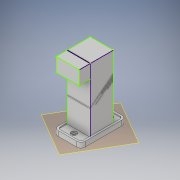
# Autodesk Inventor part: detector curvament fil
Saved by Autodesk Inventor 2019 (Build 230136000, 136)
## iProperties
Created: 2018-08-06
Part Number: detector curvament fil
Material: Genérico
Document SubType Name: Modeling
Designer: Albert Garangou Culebras
Density: 1 g/cm^3
Appearance: Valor por defecto
Mass: 54.1896 g
Surface Area: 120.446 cm^2
Volume: 54.1896 cm^3
Author: Albert Garangou Culebras
Title: suport detector curvament fil
Comments: Falta fer una possible guia per amagar el cable (dins la paret o a fora).
Autodesk Inventor part; units mm, degrees
ref_plane "YZ Plane" through (0, 0, 0) normal (1, 0, 0) x (0, 1, 0)
ref_plane "XZ Plane" through (0, 0, 0) normal (0, 1, 0) x (-1, 0, 0)
ref_plane "XY Plane" through (0, 0, 0) normal (0, 0, 1) x (1, 0, 0)
sketch3d "estructura"
sketch "base" plane through (0, 0, 0) normal (0, 1, 0) x (-1, 0, 0)
  line L0 (25, 0) -> (25, -25)
  line L1 (25, -25) -> (0, -25)
  line L2 (0, -25) -> (0, 0)
  line L3 (0, 0) -> (25, 0)
  line L4 (25, 0) -> (0, 0)
  line L5 (0, 0) -> (0, -25)
  line L6 (0, -25) -> (25, -25)
  line L7 (25, -25) -> (25, 0)
  constraints: 16 end point, 3 parallel, 1 horizontal, 1 perpendicular
sketch "Boceto4" plane through (0, 0, 0) normal (0, 0, 1) x (1, 0, 0)
  line L0 (-25, 75) -> (0, 75)
  line L1 (0, 75) -> (0, 60)
  line L2 (0, 60) -> (-25, 60)
  line L3 (-25, 60) -> (-25, 75)
  line L4 (-25, 75) -> (0, 75)
  point P0 (0, 0)
  constraints: 10 end point, 3 equal length, 1 horizontal, 1 perpendicular
extrude "suport" add sketch "Boceto4" along normal blind 12
extrude "cos" add sketch "base" along normal blind 75
sketch "borera" plane through (0, 0, 0) normal (0, -1, 0) x (1, 0, 0)
  line L0 (-25, -37) -> (0, -37)
  line L1 (-25, -25) -> (-25, 0) projected
  line L2 (0, 12) -> (-25, 12)
  line L3 (3, -24) -> (3, -37)
  line L4 (3, -37) -> (0, -37)
  line L5 (0, 12) -> (3, 12)
  line L6 (3, 12) -> (3, -24)
  line L7 (-25, -37) -> (-28, -37)
  line L8 (-25, 12) -> (-28, 12)
  line L9 (-28, 12) -> (-28, -37)
  point P0 (0, 0)
  point P1 (-25, -24)
  constraints: 18 end point, 3 horizontal, 2 perpendicular
extrude "borera?" add sketch "borera" against normal blind 7.5
sketch "LLOSA" plane through (0, 7.5, 0) normal (0, 1, 0) x (1, 0, 0)
  line L0 (0, -10) -> (-25, -10)
  line L1 (0, 35) -> (-25, 35)
  line L2 (0, -10) -> (0, 35)
  line L3 (-25, -10) -> (-25, 35)
  point P0 (0, 0)
  constraints: 8 end point, 1 perpendicular
sketch "Boceto7" plane through (3, 0, 12) normal (1, 0, 0) x (0, 0, -1)
  line L0 (0, 7.5) -> (49, 7.5)
  line L1 (49, 7.5) -> (49, 0)
  line L2 (49, 0) -> (0, 0)
  line L3 (0, 0) -> (0, 7.5)
  point P0 (12, 0)
  constraints: 8 end point, 2 parallel, 1 horizontal, 1 perpendicular
extrude "redimensió costat 2" cut sketch "Boceto7" against normal blind 1
sketch "Boceto8" plane through (-28, 0, -37) normal (-1, 0, 0) x (0, 0, 1)
  line L0 (49, 0) -> (49, 7.5) projected
  line L1 (0, 0) -> (0, 7.5) projected
  line L2 (49, 7.5) -> (0, 7.5)
  line L3 (0, 7.5) -> (0, 0)
  line L4 (0, 0) -> (49, 0)
  line L5 (49, 0) -> (49, 7.5)
  point P0 (37, 0)
  constraints: 8 end point, 2 parallel, 1 horizontal, 1 perpendicular
extrude "redimensió costat" cut sketch "Boceto8" against normal blind 1
extrude "foradar interior borera" cut sketch "LLOSA" against normal blind 1
sketch "rodons interns" plane through (0, 7.5, 0) normal (0, 1, 0) x (1, 0, 0)
  line L0 (-25, 35) -> (0, 35) projected
  line L1 (2, 35) -> (-2.5, 35)
  line L2 (-25, 35) -> (0, 35) projected
  line L3 (2, 37) -> (2, 32.5)
  line L4 (2, -12) -> (2, 37) projected
  circle A0 centre (-2.5, 32.5) radius 2.5
  circle A1 centre (-22.5, 32.5) radius 2.5
  line L5 (2, -12) -> (-2.5, -12)
  line L6 (-2.5, -12) -> (-2.5, -7.5)
  line L7 (-2.5, -7.5) -> (2, -7.5)
  line L8 (2, -7.5) -> (2, -12)
  line L9 (-27, -12) -> (-22.5, -12)
  line L10 (-22.5, -12) -> (-22.5, -7.5)
  line L11 (-22.5, -7.5) -> (-27, -7.5)
  line L12 (-27, -7.5) -> (-27, -12)
  circle A2 centre (-22.5, -7.5) radius 2.5
  line L13 (0, -10) -> (-25, -10) projected
  line L14 (-22.5, -10) -> (-25, -10)
  line L15 (-25, -10) -> (-25, -7.5)
  line L16 (-25, -10) -> (-25, 0) projected
  arc A3 (-25, -7.5) -> (-22.5, -10) centre (-22.5, -7.5) ccw
  circle A4 centre (-2.5, -7.5) radius 2.5
  arc A5 (-2.5, -10) -> (0, -7.5) centre (-2.5, -7.5) ccw
  line L17 (0, 0) -> (0, -10) projected
  line L18 (0, -7.5) -> (0, -10)
  line L19 (0, -10) -> (-2.5, -10)
  line L20 (-2.5, 35) -> (0, 35)
  line L21 (0, 35) -> (0, 25) projected
  arc A6 (0, 32.5) -> (-2.5, 35) centre (-2.5, 32.5) ccw
  arc A7 (-22.5, 35) -> (-25, 32.5) centre (-22.5, 32.5) ccw
  line L22 (-22.5, 35) -> (-25, 35)
  arc A8 (-22.5, 35) -> (-25, 32.5) centre (-22.5, 32.5) ccw
  line L23 (-25, 35) -> (-25, 32.5)
  line L24 (-25, 25) -> (-25, 35) projected
  arc A9 (-22.5, 35) -> (-25, 32.5) centre (-22.5, 32.5) ccw
  line L25 (-25, 32.5) -> (-25, 35)
  point P0 (-27, 37)
  dimension "d73" = 4.5
  dimension "d74" = 4.5
  dimension "d77" = 4.5
  dimension "d78" = 4.5
  constraints: 36 end point, 20 point on circle, 10 centre point, 7 tangent, 6 point on line, 5 collinear, 5 concentric, 4 parallel, 3 horizontal, 2 coincident, 2 perpendicular, 1 vertical
  measures "d73" distance of L1.start L1.end
  measures "d74" distance of L3.start L3.end
  measures "d77" distance of L6.end L7.end
  measures "d78" distance of L5.end L6.end
fillet "arrodoniment costats ext" radius 4.5 4 edges at (2, 3.75, -37) (-27, 3.75, -37) (2, 3.75, 12) (-27, 3.75, 12)
extrude "costats" add sketch "rodons interns" against normal blind 1 contours L0 A1 L23 | L0 L21 A0 | L17 L13 A4 | L13 L15 A2
sketch "cargols" plane through (0, 6.5, 0) normal (0, 1, 0) x (1, 0, 0)
  line L0 (0, 32.5) -> (0, 25) projected
  line L1 (-25, 25) -> (-25, 0) projected
  line L2 (-25, 0) -> (-25, -10)
  line L3 (-2.5, -10) -> (-22.5, -10) projected
  line L4 (-2.5, -10) -> (-25, -10)
  line L5 (-25, -7.5) -> (-25, 32.5) projected
  line L6 (0, 32.5) -> (0, -7.5) projected
  line L7 (-25, 25) -> (-25, 35.3997)
  line L8 (-22.5, 35) -> (-25, 35)
  line L9 (-25, 35) -> (-25, 25)
  circle A0 centre (-16.67, 30) radius 3
  circle A1 centre (-8.34, 30) radius 3
  line L10 (-25, -10) -> (-25, 0)
  circle A2 centre (-12.5, -5) radius 3
  point P0 (0, 0)
  dimension "d118" = 6
  dimension "d119" = 6
  dimension "d121" = 6
  constraints: 12 end point, 3 centre point, 3 vertical, 2 perpendicular, 2 point on line, 1 collinear
  measures "d118" diameter of A0
  measures "d119" diameter of A1
  measures "d121" diameter of A2
sketch "Boceto11" plane through (-25, 75, 12) normal (0, 1, 0) x (1, 0, 0)
  line L0 (0, 12) -> (25, 12) projected
  line L1 (25, 44.5) -> (25, 37) projected
  line L2 (0, 12) -> (25, 12)
  line L3 (25, 12) -> (25, 37)
  line L4 (25, 37) -> (0, 37)
  line L5 (0, 37) -> (0, 12)
  constraints: 8 end point, 2 parallel, 1 horizontal, 1 perpendicular
extrude "arreglo altura" add sketch "Boceto11" against normal blind 75
sketch "Boceto19" plane through (0, 0, 0) normal (0, -1, 0) x (1, 0, 0)
  line L0 (0, 12) -> (-25, 12) projected
  line L1 (-23, 12) -> (-2, 12)
  line L2 (2, -32.5) -> (2, 7.5) projected
  line L3 (2, 8) -> (2, -32.5)
  line L4 (-2.5, -37) -> (-22.5, -37) projected
  line L5 (-2.5, -37) -> (-22.5, -37)
  line L6 (-27, 7.5) -> (-27, -32.5) projected
  line L7 (-27, -32.5) -> (-27, 7.5)
  line L8 (-25, -25) -> (0, -25) projected
  line L9 (-25, 0) -> (0, 0)
  line L10 (0, 0) -> (0, -25)
  line L11 (0, -25) -> (-25, -25)
  line L12 (-25, -25) -> (-25, 0)
  point P0 (-22.5, 12)
  constraints: 16 end point, 2 collinear, 2 horizontal, 2 parallel, 2 point on line, 1 perpendicular
extrude "Extrusión11" cut sketch "Boceto19" against normal blind 1
sketch "Boceto 3D3"
ref_plane "Plano de trabajo2" through (-6.2123, 1, -23.1029) normal (0, 1, 0) x (0.8632815, 0, 0.5047227)
split "Dividir1" plane through (-6.2123, 1, -23.1029) removes the side toward (0, -1, 0)
sketch "redimensió alt" plane through (0, 7.5, 0) normal (0, 1, 0) x (1, 0, 0)
  line L0 (-3, 35) -> (-22.5, 35)
  line L1 (-22.5, 35) -> (-2.5, 35) projected
  arc A0 (-22.5, 35) -> (-25, 32.5) centre (-22.5, 32.5) ccw projected
  arc A1 (-22.5, 35) -> (-25, 32.5) centre (-22.5, 32.5) ccw
  line L2 (-25, 32.5) -> (-25, -7.5)
  line L3 (-2.5, -10) -> (-22.5, -10) projected
  arc A2 (-25, -7.5) -> (-22.5, -10) centre (-22.5, -7.5) ccw
  line L4 (-2.5, -10) -> (-22.5, -10) projected
  line L5 (-22.5, -10) -> (-2.5, -10)
  arc A3 (-2.5, -10) -> (0, -7.5) centre (-2.5, -7.5) ccw
  arc A4 (0, 32.5) -> (-2.5, 35) centre (-2.5, 32.5) ccw projected
  line L6 (0, -7.5) -> (0, 32.5)
  line L7 (0, 32.5) -> (0, 25) projected
  line L8 (-2.5, 37) -> (-22.5, 37) projected
  line L9 (-2.5714, 37) -> (-22.5, 37)
  line L10 (-2.5, 37) -> (-22.5, 37) projected
  arc A5 (-22.5, 37) -> (-27, 32.5) centre (-22.5, 32.5) ccw projected
  arc A6 (-22.5, 37) -> (-27, 32.5) centre (-22.5, 32.5) ccw
  line L11 (-27, 32.5) -> (-27, -7.5) projected
  line L12 (-27, 32.5) -> (-27, -7.5)
  arc A7 (-27, -7.5) -> (-22.5, -12) centre (-22.5, -7.5) ccw
  arc A8 (-27, -7.5) -> (-22.5, -12) centre (-22.5, -7.5) ccw projected
  line L13 (-22.5, -12) -> (-2.5714, -12)
  line L14 (2, -7.5) -> (2, 32.5) projected
  line L15 (2, -7.5) -> (2, 32.5)
  arc A9 (2, 32.5) -> (-2.5, 37) centre (-2.5, 32.5) ccw
  arc A10 (-2.5, -12) -> (2, -7.5) centre (-2.5, -7.5) ccw projected
  arc A11 (-2.5, -12) -> (2, -7.5) centre (-2.5, -7.5) ccw
  line L16 (0, 0) -> (0, -7.5) projected
  arc A12 (-2.5, -10) -> (0, -7.5) centre (-2.5, -7.5) ccw
  arc A13 (-2.5, -12) -> (2, -7.5) centre (-2.5, -7.5) ccw
  arc A14 (-22.5, 35) -> (-25, 32.5) centre (-22.5, 32.5) ccw
  arc A15 (-22.5, 37) -> (-27, 32.5) centre (-22.5, 32.5) ccw
  arc A16 (0, 32.5) -> (-2.5, 35) centre (-2.5, 32.5) ccw
  line L17 (-2.5, 35) -> (-22.5, 35)
  arc A17 (-22.5, 35) -> (-25, 32.5) centre (-22.5, 32.5) ccw projected
  arc A18 (-22.5, 35) -> (-25, 32.5) centre (-22.5, 32.5) ccw
  arc A19 (-22.5, 37) -> (-27, 32.5) centre (-22.5, 32.5) ccw
  arc A20 (-25, -7.5) -> (-22.5, -10) centre (-22.5, -7.5) ccw projected
  arc A21 (-25, -7.5) -> (-22.5, -10) centre (-22.5, -7.5) ccw
  arc A22 (-27, -7.5) -> (-22.5, -12) centre (-22.5, -7.5) ccw
  arc A23 (-2.5, -10) -> (0, -7.5) centre (-2.5, -7.5) ccw projected
  arc A24 (-2.5, -10) -> (0, -7.5) centre (-2.5, -7.5) ccw
  line L18 (0, 0) -> (-25, 0) projected
  line L19 (-25, 0) -> (-25, -7.5)
  line L20 (-22.5, -10) -> (-2.5, -10)
  line L21 (0, -7.5) -> (0, 0)
  line L22 (0, 32.5) -> (0, 0)
  arc A25 (0, 32.5) -> (-2.5, 35) centre (-2.5, 32.5) ccw projected
  line L23 (-2.5, 35) -> (-22.5, 35)
  line L24 (-22.5, 37) -> (-2.5, 37)
  line L25 (2, 32.5) -> (2, -7.5)
  line L26 (-22.5, -10) -> (-2.5, -10)
  line L27 (-22.5, -12) -> (-2.5, -12) projected
  line L28 (-22.5, -12) -> (-2.5, -12) projected
  line L29 (-2.5, -12) -> (-22.5, -12)
  line L30 (-27, -7.5) -> (-27, 32.5)
  line L31 (-25, 25) -> (-25, 32.5) projected
  line L32 (-25, 32.5) -> (-25, -7.5)
  line L33 (-22.5, 35) -> (-3, 35)
  arc A26 (2, 32.5) -> (-2.5, 37) centre (-2.5, 32.5) ccw projected
  line L34 (-2.5, 37) -> (-22.5, 37)
  constraints: 44 end point, 35 point on circle, 31 tangent, 17 centre point, 6 horizontal, 5 collinear, 5 perpendicular, 5 vertical, 4 concentric, 1 parallel
sketch "redimensió 2" plane through (0, 6.5, 0) normal (0, 1, 0) x (1, 0, 0)
  line L0 (0, 32.5) -> (0, 25) projected
  line L1 (-25, 25) -> (-25, 32.5) projected
  line L2 (0, 25) -> (-25, 25)
  line L3 (-25, 25) -> (-25, 32.5)
  line L4 (-22.5, 35) -> (-2.5, 35) projected
  arc A0 (-22.5, 35) -> (-25, 32.5) centre (-22.5, 32.5) ccw
  line L5 (-22.5, 35) -> (-2.5, 35)
  line L6 (0, 32.5) -> (0, 25)
  line L7 (0, 0) -> (-25, 0) projected
  line L8 (0, 0) -> (-25, 0)
  line L9 (-25, -7.5) -> (-25, 0) projected
  line L10 (-25, 0) -> (-25, -7.5)
  arc A1 (-25, -7.5) -> (-22.5, -10) centre (-22.5, -7.5) ccw projected
  arc A2 (-25, -7.5) -> (-22.5, -10) centre (-22.5, -7.5) ccw
  line L11 (-2.5, -10) -> (-22.5, -10) projected
  line L12 (-22.5, -10) -> (-2.5, -10)
  line L13 (0, 0) -> (0, -7.5) projected
  arc A3 (-2.5, -10) -> (0, -7.5) centre (-2.47, -7.53) ccw
  line L14 (0, -7.5) -> (0, 0)
  line L15 (-25, 0) -> (0, 0)
  line L16 (0, -7.5) -> (0, 0)
  arc A4 (-2.5, -10) -> (0, -7.5) centre (-2.5, -7.5) ccw projected
  line L17 (-2.5, -10) -> (-22.5, -10)
  arc A5 (-25, -7.5) -> (-22.5, -10) centre (-22.5, -7.5) ccw
  arc A6 (-2.5, -10) -> (0, -7.5) centre (-2.25, -7.75) ccw
  line L18 (0, 32.5) -> (0, 25) projected
  arc A7 (0, 32.5) -> (-2.5, 35) centre (-2.5, 32.5) ccw
  arc A8 (-22.5, 35) -> (-25, 32.5) centre (-22.5, 32.5) ccw
  line L19 (-22.5, 35) -> (-2.5, 35) projected
  line L20 (-22.5, 35) -> (-2.5, 35)
  line L21 (0, 32.5) -> (0, 25)
  line L22 (-25, 25) -> (-25, 32.5)
  line L23 (-27, 32.5) -> (-27, -7.5) projected
  line L24 (-25, 25) -> (0, 25) projected
  line L25 (-25, 25) -> (0, 25)
  constraints: 30 end point, 16 point on circle, 7 centre point, 6 collinear, 4 horizontal, 2 perpendicular, 2 tangent, 1 parallel, 1 point on line, 1 vertical
extrude "redimensió ext altura" cut sketch "redimensió alt" against normal blind 1
extrude "redimensió ext 2" cut sketch "redimensió 2" against normal blind 1 contours L0 L2 L1 A0 L4 A7 | L13 A4 L11 A1 L9 L7 | A3 A4
extrude "forats cargols" cut sketch "cargols" against normal blind 2.8
sketch "Boceto24" plane through (-16.67, 3.7, -30) normal (0, 1, 0) x (1, 0, 0)
  circle A0 centre (0, 0) radius 1.55
  line L0 (0, 0) -> (8.33, 0)
  circle A1 centre (8.33, 0) radius 1.55
  circle A2 centre (4.17, -35) radius 3 projected
  circle A3 centre (4.17, -35) radius 1.55
  point P0 (16.67, -30)
  dimension "d124" = 3.1
  dimension "d125" = 8.33
  dimension "d126" = 3.1
  dimension "d127" = 3.1
  constraints: 3 centre point, 2 coincident, 2 end point, 1 horizontal
  measures "d124" diameter of A0
  measures "d125" distance of L0.start L0.end
  measures "d126" diameter of A1
  measures "d127" diameter of A3
extrude "forats cargols rosca" cut sketch "Boceto24" against normal blind 5 contours A0 | A1 | A3
sketch "Boceto25" plane through (-25, 75, 12) normal (0, 1, 0) x (1, 0, 0)
  line L0 (25, 12) -> (25, 4.5) projected
  line L1 (25, 12) -> (25, 12.5)
  line L2 (25, 12) -> (25, 37) projected
  line L3 (25, 12.5) -> (25, 12)
  line L4 (25, 12) -> (25, 11.5)
  line L5 (25, 11.5) -> (0, 11.5)
  line L6 (0, 4.5) -> (0, 12) projected
  line L7 (25, 12.5) -> (0, 12.5)
  line L8 (0, 37) -> (0, 12) projected
  line L9 (0, 11.5) -> (0, 12.5)
  dimension "d130" = 0.5
  dimension "d131" = 0.5
  constraints: 12 end point, 4 point on line, 2 equal length, 2 perpendicular
  measures "d130" distance of L0.start L1.end
  measures "d131" distance of L0.start L4.end
extrude "marca dalt" cut sketch "Boceto25" against normal blind 0.5
sketch "Boceto26" plane through (0, 1, 0) normal (0, -1, 0) x (1, 0, 0)
  line L0 (-25.443, -26.1307) -> (-20.3716, -26.1307) construction
  line L1 (-20.3716, -26.1307) -> (-20.3716, -34.2106) construction
  line L2 (-20.3716, -34.2106) -> (-25.443, -34.2106) construction
  line L3 (-25.443, -34.2106) -> (-25.443, -26.1307) construction
  line L4 (-22.9236, -26.1406) -> (-23.9734, -29.1886)
  line L5 (-23.9734, -29.1886) -> (-24.4106, -29.1886)
  line L6 (-24.4106, -29.1886) -> (-25.4603, -26.1406)
  line L7 (-25.4603, -26.1406) -> (-25.0256, -26.1406)
  line L8 (-25.0256, -26.1406) -> (-24.1809, -28.6723)
  line L9 (-24.1809, -28.6723) -> (-23.3361, -26.1406)
  line L10 (-23.3361, -26.1406) -> (-22.9236, -26.1406)
  line L11 (-20.9921, -29.1886) -> (-22.479, -29.1886)
  line L12 (-22.479, -29.1886) -> (-22.479, -28.8774)
  line L13 (-22.479, -28.8774) -> (-21.9257, -28.8774)
  line L14 (-21.9257, -28.8774) -> (-21.9257, -26.8347)
  line L15 (-21.9257, -26.8347) -> (-22.479, -26.8347)
  line L16 (-22.479, -26.8347) -> (-22.479, -26.5555)
  spline S0 degree 2 poles (-22.479, -26.5555) (-22.1653, -26.5555) (-21.8689, -26.3777) (-21.8492, -26.1307) knots 0 0 0 1 2 2 2
  line L17 (-21.8492, -26.1307) -> (-21.533, -26.1307)
  line L18 (-21.533, -26.1307) -> (-21.533, -28.8774)
  line L19 (-21.533, -28.8774) -> (-20.9921, -28.8774)
  line L20 (-20.9921, -28.8774) -> (-20.9921, -29.1886)
  point P0 (0, 0)
  constraints: 2 other
extrude "num versió" cut sketch "Boceto26" against normal blind 0.8
sketch "Boceto28" plane through (-25, 60, 12) normal (-1, 0, 0) x (0, 0, 1)
  line L0 (-37, -53.5) -> (-37, 15) projected
  line L1 (-37, -7) -> (-12, -26.75)
  line L2 (-12, -53.5) -> (-12, 0) projected
  line L3 (-37, -7) -> (-37, -8)
  line L4 (-37, -8) -> (-12, -27.75)
  line L5 (-37, -8) -> (-37, -9)
  line L6 (-37, -9) -> (-37, -10)
  line L7 (-37, -10) -> (-37, -11)
  line L8 (-37, -11) -> (-37, -12)
  line L9 (-37, -12) -> (-37, -13)
  line L10 (-37, -13) -> (-37, -14)
  line L11 (-37, -14) -> (-37, -15)
  line L12 (-37, 0) -> (-12, 0)
  line L13 (-37, 0) -> (-30.75, 0)
  line L14 (-30.75, 0) -> (-24.5, 0)
  line L15 (-24.5, 0) -> (-18.25, 0)
  line L16 (-30.75, 0) -> (-30.75, -29)
  line L17 (-24.5, 0) -> (-24.5, -29)
  line L18 (-18.25, 0) -> (-18.25, -29)
  line L19 (-37, -9) -> (-24.5, -19)
  line L20 (-37, -10) -> (-24.5, -20)
  line L21 (-24.5, -19) -> (-24.5, -20)
  line L22 (-37, -11) -> (-18.25, -26)
  line L23 (-18.25, -26) -> (-18.25, -27)
  line L24 (-18.25, -27) -> (-37, -12)
  line L25 (-37, -13) -> (-30.75, -18)
  line L26 (-30.75, -18) -> (-30.75, -19)
  line L27 (-37, -14) -> (-30.75, -19)
  line L28 (-12, -27.75) -> (-12, -26.75)
  point P0 (-12, -60)
  dimension "d136" = 1
  dimension "d137" = 1
  dimension "d138" = 1
  dimension "d139" = 1
  dimension "d140" = 1
  dimension "d141" = 1
  dimension "d142" = 1
  dimension "d143" = 1
  dimension "d144" = 6.25
  dimension "d145" = 6.25
  dimension "d146" = 6.25
  dimension "d147" = 1
  constraints: 54 end point, 8 point on line, 5 vertical, 3 parallel, 2 midpoint, 1 horizontal, 10 other
  measures "d136" distance of L1.start L3.end
  measures "d137" distance of L3.end L5.end
  measures "d138" distance of L5.end L6.end
  measures "d139" distance of L6.end L7.end
  measures "d140" distance of L7.end L8.end
  measures "d141" distance of L8.end L9.end
  measures "d142" distance of L9.end L10.end
  measures "d143" distance of L10.end L11.end
  measures "d144" distance of L12.start L13.end
  measures "d145" distance of L13.end L14.end
  measures "d146" distance of L14.end L15.end
  measures "d147" distance of L22.end L23.end
extrude "Extrusión22" cut sketch "Boceto28" against normal blind 0.8 contours L0 L25 L16 L27 | L0 L22 L16 L24 | L16 L22 L17 L24 | L0 L19 L16 L20 | L17 L22 L18 L24 | L16 L19 L17 L20 | L0 L1 L16 L4 | L16 L1 L17 L4 | L18 L1 L2 L4 | L4 L17 L1 L18
sketch "Boceto29" plane through (-25, 60, 0) normal (0, 0, 1) x (1, 0, 0)
  line L0 (0, -7) -> (0, -26.75) projected
  line L1 (0, -26.75) -> (25, -26.75)
  line L2 (0.8, -27.75) -> (0, -27.75) projected
  line L3 (25, -26.75) -> (25, -27.75)
  line L4 (25, -53.5) -> (25, 0) projected
  line L5 (0, -26.75) -> (0, -27.75)
  line L6 (0.8, -26.75) -> (0.8, -27.75) projected
  line L7 (0.8, -27.75) -> (0.8, -26.75)
  line L8 (0.8, -26.75) -> (0.8, -27.75)
  line L9 (25, -27.75) -> (0.8, -27.75)
  line L10 (25, -53.5) -> (25, 15) projected
  line L11 (25, -26.75) -> (24.2, -26.75)
  line L12 (24.2, -26.75) -> (24.2, -27.75)
  point P0 (25, -60)
  dimension "d150" = 0.8
  constraints: 16 end point, 3 collinear, 2 perpendicular, 2 point on line, 1 horizontal, 1 parallel
  measures "d150" distance of L1.end L11.end
extrude "Extrusión23" cut sketch "Boceto29" against normal blind 0.8 contours L1 L12 L9 L6
sketch "Boceto32" plane through (0, 60, 12) normal (1, 0, 0) x (0, 0, -1)
  line L0 (37, -53.5) -> (37, 15) projected
  line L1 (37, -7) -> (12, -26.75)
  line L2 (37, -8) -> (37, -9)
  line L3 (37, -9) -> (37, -10)
  line L4 (37, -10) -> (37, -11)
  line L5 (37, -11) -> (37, -12)
  line L6 (37, -13) -> (37, -12)
  line L7 (37, -13.9375) -> (37, -13)
  line L8 (12, -53.5) -> (12, 0) projected
  line L9 (37, 0) -> (12, 0)
  line L10 (12, 0) -> (18.25, 0)
  line L11 (18.25, 0) -> (24.5, 0)
  line L12 (24.5, 0) -> (30.75, 0)
  line L13 (37, -9) -> (24.5, -18.875)
  line L14 (24.5, -18.875) -> (24.5, -19.875)
  line L15 (37, -7) -> (12, -26.75) projected
  line L16 (37, -11) -> (18.25, -25.8125)
  line L17 (18.25, -25.8125) -> (18.25, -26.8125)
  line L18 (18.25, -26.8125) -> (37, -12)
  line L19 (37, -13) -> (30.75, -17.9375)
  line L20 (30.75, -17.9375) -> (30.75, -18.9375)
  line L21 (30.75, -18.9375) -> (37, -13.9375)
  line L22 (24.5, -19.875) -> (37, -10)
  line L23 (37, -8) -> (12, -27.75)
  line L24 (12, -26.75) -> (12, -27.75) projected
  line L25 (12, -26.75) -> (12, -27.75)
  line L26 (37, -7) -> (12, -26.75)
  line L27 (37, -9) -> (24.5, -18.875)
  line L28 (24.5, -19.875) -> (24.5, -18.875)
  line L29 (24.5, -19) -> (24.5, -20) projected
  point P0 (12, -60)
  dimension "d156" = 6.25
  dimension "d157" = 6.25
  constraints: 50 end point, 3 collinear, 3 parallel, 3 point on line, 2 vertical, 1 midpoint, 1 perpendicular, 9 other
  measures "d156" distance of L8.end L10.end
  measures "d157" distance of L10.end L11.end
extrude "Extrusión24" cut sketch "Boceto32" against normal blind 0.8 contours L21 L20 L19 L0 | L18 L17 L16 L0 | L22 L14 L13 L0
sketch "Boceto33" plane through (0, 60, 12) normal (1, 0, 0) x (0, 0, -1)
  line L0 (12, -53.5) -> (12, 0) projected
  line L1 (12, -26.75) -> (37, -7)
  line L2 (37, -7) -> (37, -8)
  line L3 (37, -9) -> (37, 15) projected
  line L4 (37, -8) -> (12, -27.75)
  point P0 (12, -60)
  constraints: 6 end point, 1 midpoint, 1 parallel, 1 point on line
extrude "Extrusión25" cut sketch "Boceto33" against normal blind 0.8 fills toward (24.531, -16.9142) open curves L1 L2 L4
sketch "Boceto34" plane through (-24.2, 32.25, -0.8) normal (1, 0, 0) x (0, 0, -1)
  line L0 (-0.8, 0) -> (24.2, 19.75) projected
  line L1 (0, 0) -> (0, 0.632) projected
  line L2 (0, 0.632) -> (0, 0)
  line L3 (0, 0) -> (-0.8, 0)
  line L4 (-0.8, 0) -> (0, 0.632)
  point P0 (-0.8, -32.25)
  constraints: 6 end point, 1 collinear, 1 perpendicular, 1 point on line
extrude "Extrusión26" add sketch "Boceto34" along normal blind 23.8
sketch "Boceto35" plane through (-24.2, 60, 12) normal (-1, 0, 0) x (0, 0, 1)
  line L0 (-12.8, -27.118) -> (-12.8, -26.75) projected
  line L1 (-12.8, -27.118) -> (-12.8, -26.75)
  line L2 (-12.8, -6.75) -> (-12.8, -26.118)
  line L3 (-37, -7) -> (-12, -26.75) projected
  line L4 (-12.8, -26.75) -> (-12.8, -26.118)
  line L5 (-12.8, -26.75) -> (-12, -26.75) projected
  line L6 (-12.8, -26.118) -> (-12, -26.75)
  line L7 (-12, -26.75) -> (-12.8, -26.75)
  point P0 (-12, -60)
  constraints: 10 end point, 3 collinear, 2 point on line
extrude "Extrusión27" cut sketch "Boceto35" against normal blind 97.95
